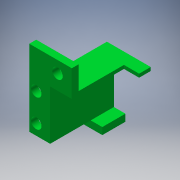
# Autodesk Inventor part: MotorMount
Saved by Autodesk Inventor 2016 (Build 200138000, 138)
## iProperties
Created: 2014-06-07
Part Number: MotorMount
Material: Generic
Document SubType Name: Modeling
Designer: Erin
Density: 1 g/cm^3
Appearance: Default
Author: Erin
Autodesk Inventor part; units mm, degrees
ref_plane "YZ Plane" through (0, 0, 0) normal (1, 0, 0) x (0, 1, 0)
ref_plane "XZ Plane" through (0, 0, 0) normal (0, 1, 0) x (-1, 0, 0)
ref_plane "XY Plane" through (0, 0, 0) normal (0, 0, 1) x (1, 0, 0)
sketch "Sketch1" plane through (0, 0, 0) normal (0, 1, 0) x (-1, 0, 0)
  line L0 (-9.45, 13.9) -> (9.45, 13.9)
  line L1 (9.45, 13.9) -> (9.45, 12.4)
  line L2 (9.45, 12.4) -> (-9.45, 12.4)
  line L3 (-9.45, 12.4) -> (-9.45, 13.9)
  line L4 (9.45, 12.4) -> (6.45, 12.4)
  line L5 (6.45, 12.4) -> (6.45, -9)
  line L6 (6.45, -9) -> (9.45, -9)
  line L7 (9.45, -9) -> (9.45, 12.4)
  line L8 (-9.45, 12.4) -> (-7.95, 12.4)
  line L9 (-7.95, 12.4) -> (-7.95, -9)
  line L10 (-7.95, -9) -> (-9.45, -9)
  line L11 (-9.45, -9) -> (-9.45, 12.4)
  line L12 (-7.95, -9) -> (-9.45, -9)
  line L13 (-9.45, -9) -> (-9.45, -12)
  line L14 (-9.45, -12) -> (-7.95, -12)
  line L15 (-7.95, -12) -> (-7.95, -9)
  line L16 (1.45, -9) -> (9.45, -9)
  line L17 (9.45, -9) -> (9.45, -12)
  line L18 (9.45, -12) -> (1.45, -12)
  line L19 (1.45, -12) -> (1.45, -9)
  line L20 (-9.45, -12) -> (-7.95, -12)
  line L21 (9.45, -12) -> (6.45, -12)
  line L22 (-7.95, -12) -> (-4.95, -12)
  line L23 (-4.95, -12) -> (-4.95, -9)
  line L24 (-4.95, -9) -> (-7.95, -9)
  line L25 (-7.95, -9) -> (-7.95, -12)
  point P0 (0, 0)
  point P1 (0, 12.4)
  dimension "d0" = 1.5
  dimension "d1" = 3
  dimension "d2" = 1.5
  dimension "d3" = 3
  dimension "d4" = 3
  dimension "d5" = 0
  dimension "d6" = 5
  dimension "d7" = 14.4
  dimension "d8" = 21.4
  dimension "d9" = 21.4
  dimension "d12" = 0
  dimension "d13" = 0
  dimension "d38" = 3
  constraints: 52 end point, 12 parallel, 8 horizontal, 6 perpendicular, 1 collinear, 1 midpoint, 1 vertical alignment
  measures "d0" distance of L0.end L1.end
  measures "d1" distance of L5.end L6.end
  measures "d2" distance of L9.end L10.end
  measures "d3" distance of L14.end L12.start
  measures "d4" distance of L18.end L16.start
  measures "d5" distance between parallel lines of L15 L9
  measures "d6" distance between parallel lines of L5 L19
  measures "d7" distance between parallel lines of L5 L9
  measures "d8" distance between parallel lines of L16 L2
  measures "d9" distance between parallel lines of L12 L2
  measures "d12" distance between parallel lines of L11 L13
  measures "d13" distance between parallel lines of L7 L17
  measures "d38" distance of L24.end L23.end
extrude "Extrusion1" add sketch "Sketch1" along normal blind 10 contours L0 L1 L2 L3 | L7 L6 L5 L2 | L17 L18 L19 L16 L6
sketch "Sketch8" plane through (0, 0, 0) normal (0, -1, 0) x (1, 0, 0)
  line L0 (2.9056, 13.9) -> (14.45, 13.9)
  line L1 (14.45, 13.9) -> (14.45, -22.6)
  line L2 (14.45, -22.6) -> (2.9056, -22.6)
  line L3 (2.9056, -22.6) -> (2.9056, 13.9)
  line L4 (-9.45, 13.9) -> (9.45, 13.9) projected
  point P0 (0, 0)
  constraints: 8 end point, 2 parallel, 1 collinear, 1 horizontal, 1 perpendicular
extrude "Extrusion6" cut sketch "Sketch8" against normal blind 5
sketch "Sketch9" plane through (0, 0, 0) normal (0, -1, 0) x (1, 0, 0)
  line L0 (2.9056, 12.4) -> (2.9056, 13.9) projected
  line L1 (-9.45, 13.9) -> (2.9056, 13.9) projected
  line L2 (-9.45, 13.9) -> (-9.45, -12) projected
  line L3 (-9.45, -12) -> (-1.45, -12) projected
  line L4 (-1.45, -12) -> (-1.45, -9) projected
  line L5 (-1.45, -9) -> (-6.45, -9) projected
  line L6 (-6.45, 12.4) -> (-6.45, -9) projected
  line L7 (2.9056, 12.4) -> (-6.45, 12.4) projected
  line L8 (-6.45, -9) -> (-1.45, -9) projected
  line L9 (-9.45, -12) -> (-9.45, 13.9) projected
  line L10 (-6.45, -9) -> (-9.45, -9)
  line L11 (-9.45, -9) -> (-9.45, 12.4)
  line L12 (-9.45, 12.4) -> (-6.45, 12.4)
  line L13 (-6.45, 12.4) -> (-6.45, -9)
  point P0 (0, 0)
  constraints: 8 end point, 2 parallel, 1 horizontal, 1 perpendicular, 1 point on line
extrude "Extrusion7" add sketch "Sketch9" along normal blind 17.5 contours L6 L10 L2 L12
sketch "Sketch10" plane through (-9.45, 0, 13.9) normal (-1, 0, 0) x (0, 0, 1)
  line L0 (-22.9, -17.5) -> (-1.5, -17.5) projected
  line L1 (-1.5, 0) -> (-1.5, -17.5) projected
  line L2 (-22.9, -17.5) -> (-1.5, -17.5)
  line L3 (-1.5, -17.5) -> (-1.5, -14.5)
  line L4 (-1.5, -14.5) -> (-22.9, -14.5)
  line L5 (-22.9, -14.5) -> (-22.9, -17.5)
  point P0 (-13.9, 0)
  dimension "d41" = 3
  constraints: 8 end point, 2 parallel, 1 horizontal, 1 perpendicular, 1 point on line
  measures "d41" distance of L3.end L2.end
extrude "Extrusion8" add sketch "Sketch10" along normal blind 6
sketch "Sketch11" plane through (-9.45, -14.5, 12.4) normal (0, 1, 0) x (1, 0, 0)
  line L0 (0, 21.4) -> (0, 0) projected
  line L1 (0, 21.4) -> (-6, 21.4) projected
  line L2 (-6, 0) -> (-6, 21.4) projected
  line L3 (0, 0) -> (-6, 0) projected
  line L4 (3, 21.4) -> (-6, 21.4) projected
  line L5 (-3, 21.4) -> (-3, 0) construction
  circle A0 centre (-3, 4.7) radius 2.25
  circle A1 centre (-3, 16.7) radius 2.25
  line L6 (-6, 0) -> (-6, 21.4) projected
  line L7 (-6, 10.7) -> (0, 10.7) construction
  point P0 (9.45, 12.4)
  dimension "d44" = 4.5
  dimension "d45" = 4.5
  dimension "d50" = 6
  dimension "d51" = 6
  constraints: 4 end point, 3 midpoint, 3 point on line, 2 centre point
  measures "d44" diameter of A0
  measures "d45" diameter of A1
  measures "d50" distance from line of A1.centre L7
  measures "d51" distance from line of A0.centre L7
extrude "Extrusion9" cut sketch "Sketch11" against normal blind 3 contours A0 | A1
sketch "Sketch12" plane through (0, 0, 0) normal (0, -1, 0) x (1, 0, 0)
  line L0 (-9.45, 12.4) -> (-6.45, 12.4) projected
  line L1 (2.9056, 12.4) -> (-6.45, 12.4) projected
  line L2 (2.9056, 12.4) -> (2.9056, 13.9) projected
  line L3 (-9.45, 13.9) -> (2.9056, 13.9) projected
  line L4 (-9.45, 13.9) -> (-9.45, 12.4) projected
  point P0 (0, 0)
extrude "Extrusion10" add sketch "Sketch12" along normal blind 17.5
sketch "Sketch13" plane through (-9.45, 10, 13.9) normal (0, 0, 1) x (1, 0, 0)
  line L0 (12.3556, -27.5) -> (12.3556, -5) projected
  line L1 (12.3556, -5) -> (18.9, -5) projected
  line L2 (18.9, -5) -> (18.9, 0) projected
  line L3 (0, 0) -> (18.9, 0) projected
  line L4 (0, -27.5) -> (0, 0) projected
  line L5 (12.3556, -27.5) -> (0, -27.5) projected
  line L6 (12.3556, -5) -> (12.3556, -27.5) projected
  line L7 (0, -27.5) -> (0, 0) projected
  line L8 (12.3556, -27.5) -> (0, -27.5)
  line L9 (0, -27.5) -> (0, -24.5)
  line L10 (0, -24.5) -> (12.3556, -24.5)
  line L11 (12.3556, -24.5) -> (12.3556, -27.5)
  point P0 (9.45, -10)
  dimension "d54" = 3
  constraints: 8 end point, 2 parallel, 1 horizontal, 1 perpendicular, 1 point on line
  measures "d54" distance of L8.end L9.end
extrude "Extrusion11" add sketch "Sketch13" along normal blind 10 contours L5 L4 L10 L0
sketch "Sketch14" plane through (-9.45, -14.5, 13.9) normal (0, 1, 0) x (1, 0, 0)
  line L0 (0, 0) -> (12.3556, 0) projected
  line L1 (0, 0) -> (0, -10) projected
  line L2 (12.3556, -10) -> (0, -10) projected
  line L3 (12.3556, 0) -> (12.3556, -10) projected
  circle A0 centre (6.1778, -5) radius 2.25
  point P0 (9.45, 13.9)
  dimension "d57" = 4.5
  constraints: 1 centre point
  measures "d57" diameter of A0
extrude "Extrusion12" cut sketch "Sketch14" against normal blind 3 contours A0
sketch "Sketch15" plane through (-9.45, 0, -12) normal (-1, 0, 0) x (0, 0, 1)
  line L0 (3, -14.5) -> (24.4, -14.5) projected
  line L1 (24.4, -17.5) -> (24.4, -14.5) projected
  line L2 (24.4, -17.5) -> (35.9, -17.5) projected
  line L3 (35.9, -14.5) -> (35.9, -17.5) projected
  line L4 (25.9, -14.5) -> (35.9, -14.5) projected
  line L5 (25.9, -14.5) -> (25.9, 10) projected
  line L6 (0, 10) -> (25.9, 10) projected
  line L7 (0, 0) -> (0, 10) projected
  line L8 (3, 0) -> (0, 0) projected
  line L9 (3, 0) -> (3, -14.5) projected
  line L10 (24.4, -17.5) -> (35.9, -17.5) projected
  line L11 (24.4, -17.5) -> (24.4, -14.5) projected
  line L12 (35.9, -17.5) -> (24.4, -17.5)
  line L13 (24.4, -17.5) -> (24.4, -14.5)
  line L14 (24.4, -14.5) -> (35.9, -14.5)
  line L15 (35.9, -14.5) -> (35.9, -17.5)
  point P0 (12, 0)
  constraints: 8 end point, 2 parallel, 1 horizontal, 1 perpendicular
extrude "Extrusion13" add sketch "Sketch15" along normal blind 6 contours L14 L4 L3 L2 L1
sketch "Sketch16" plane through (0, -17.5, 0) normal (0, -1, 0) x (1, 0, 0)
  circle A0 centre (-3.2722, 18.9) radius 2.25 projected
  circle A1 centre (-12.45, 7.7) radius 2.25 projected
  circle A2 centre (-12.45, -4.3) radius 2.25 projected
  line L0 (-6.45, -9) -> (-15.45, -9) projected
  line L1 (-6.45, -9) -> (-6.45, 12.4) projected
  line L2 (-6.45, 12.4) -> (2.9056, 12.4) projected
  line L3 (2.9056, 12.4) -> (2.9056, 23.9) projected
  line L4 (2.9056, 23.9) -> (-15.45, 23.9) projected
  line L5 (-15.45, -9) -> (-15.45, 23.9) projected
  point P0 (0, 0)
equation "\"sp\" = 0.4"
body "Solid1"
